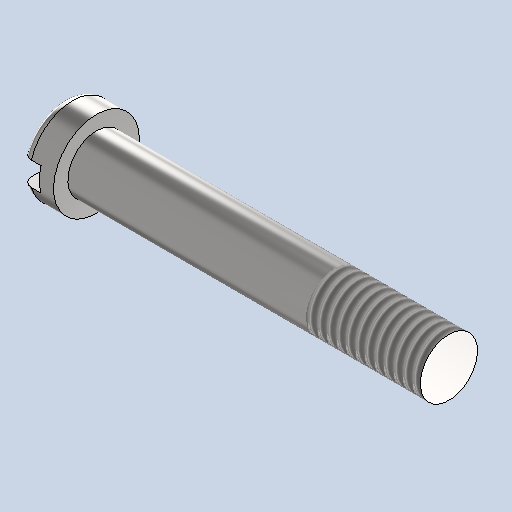
# Autodesk Inventor part: screw
Saved by Autodesk Inventor 2025 (Build 290162010, 162A)
## iProperties
Created: 2024-06-06
Part Number: screw
Material: Steel, Cast
Document SubType Name: Modeling
Designer: ffogue
Density: 7.85 g/cm^3
Appearance: Semi-Polished
Author: ffogue
Autodesk Inventor part; units mm, degrees
ref_plane "YZ Plane" through (0, 0, 0) normal (1, 0, 0) x (0, 1, 0)
ref_plane "XZ Plane" through (0, 0, 0) normal (0, 1, 0) x (-1, 0, 0)
ref_plane "XY Plane" through (0, 0, 0) normal (0, 0, 1) x (1, 0, 0)
sketch "Skizze1" plane through (0, 0, 0) normal (0, 1, 0) x (-1, 0, 0)
  line L0 (0, 0) -> (0, 4.5)
  line L1 (0, 4.5) -> (-3.5, 4.5)
  line L2 (-3.5, 4.5) -> (-3.5, 3)
  line L3 (-3.5, 3) -> (-40.5, 3)
  line L4 (-40.5, 3) -> (-40.5, 0)
  line L5 (-40.5, 0) -> (0, 0)
  dimension "d0" = 3.5
  dimension "d1" = 6
  dimension "d2" = 9
  dimension "d3" = 37
  constraints: 12 end point, 5 perpendicular, 1 vertical
  measures "d0" distance between parallel lines of L2 L0
  measures "d1" diameter of L3 L5
  measures "d2" diameter of L1 L5
  measures "d3" distance from line of L2.end L4
revolve "Umdrehung1" add sketch "Skizze1" angle 360 about axis through (40.5, 0, 0) along (-1, 0, 0)
thread "Gewinde1" size "M6x1" class "6g" standard "ISO Metric profile" length 12
sketch "Skizze2" plane through (0, 0, 0) normal (-1, 0, 0) x (0, 0, 1)
  line L0 (1.25, 4.3229) -> (1.25, -4.3229)
  line L1 (-1.25, -4.3229) -> (-1.25, 4.3229)
  circle A0 centre (0, 0) radius 4.5 projected
  line L2 (0, 4.5) -> (0, -4.5) construction
  point P0 (0, 0)
  dimension "d7" = 2.5
  constraints: 6 end point, 4 point on circle, 2 horizontal alignment, 1 parallel, 1 other
  measures "d7" distance between parallel lines of L0 L1
extrude "Extrusion1" cut sketch "Skizze2" against normal blind 2 contours L0 A0 L1
fillet "Rundung1" radius 1 3 edges at (0, 2.7042, 3.5969) (0, -2.7042, 3.5969) (0, 0, -4.5)
